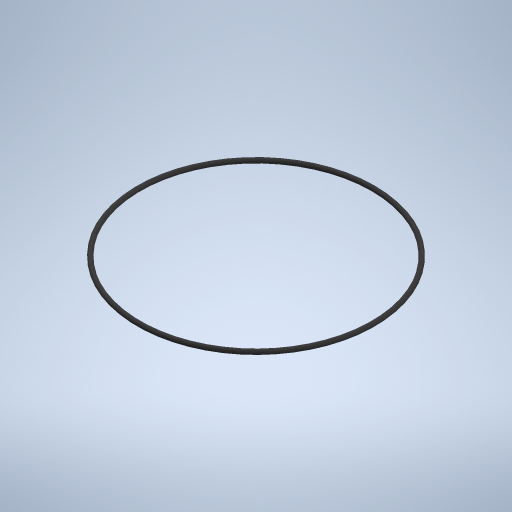
# Autodesk Inventor part: seal
Saved by Autodesk Inventor 2024 (Build 280153020, 153B)
## iProperties
Created: 2023-06-13
Part Number: seal
Material: Rubber
Document SubType Name: Modeling
Designer: OKESH
Density: 0.93 g/cm^3
Appearance: Rubber - Black
Author: OKESH
Autodesk Inventor part; units mm, degrees
ref_plane "YZ Plane" through (0, 0, 0) normal (1, 0, 0) x (0, 1, 0)
ref_plane "XZ Plane" through (0, 0, 0) normal (0, 1, 0) x (-1, 0, 0)
ref_plane "XY Plane" through (0, 0, 0) normal (0, 0, 1) x (1, 0, 0)
sketch "Sketch1" plane through (0, 0, 0) normal (1, 0, 0) x (0, 1, 0)
  circle A0 centre (0, 38.25) radius 0.75
  line L0 (0.3463, 0) -> (8.6698, 0)
  point P0 (0, 0)
  dimension "d0" = 1.5
  dimension "d1" = 38.25
  constraints: 2 end point, 1 centre point, 1 horizontal
  measures "d0" diameter of A0
  measures "d1" distance of A0.centre point (0, 0)
revolve "Revolution1" add sketch "Sketch1" angle 360 about axis through (0, 0.3463, 0) along (0, 1, 0)
body "Solid1"
